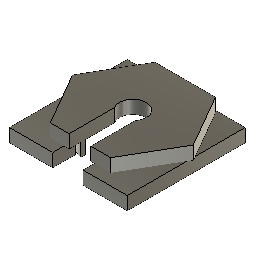
wall plug v1 v1 (Autodesk Fusion 360 design; units mm, degrees)
Autodesk Fusion 360 part; units mm, degrees
sketch "Sketch1" plane through (0, 0, 0) normal (0, 0, 1) x (1, 0, 0)
  line L0 (9.8948, 0) -> (0, 0)
  line L1 (0, 0) -> (0, 27)
  line L2 (0, 27) -> (27, 27)
  line L3 (27, 27) -> (27, 0)
  line L4 (27, 0) -> (16.8982, 0)
  circle A0 centre (13.6982, 15.0358) radius 10.55
  line L5 (9.8948, 0) -> (9.8948, 5.1952)
  line L6 (16.8982, 0) -> (16.8982, 4.9828)
  dimension "d1" = 27
  dimension "d2" = 27
  dimension "d3" = 21.1
  constraint coincident L0.end L1.start
  constraint horizontal L0
  constraint perpendicular L0 L1
  constraint perpendicular L1 L2
  constraint perpendicular L2 L3
  constraint perpendicular L3 L4
  constraint coincident A0 L5.end
  constraint perpendicular L0 L5
  constraint coincident A0 L6.end
  constraint perpendicular L4 L6
  measures "d1" distance of L0.end L1.end
  measures "d2" distance of L1.end L2.end
  measures "d3" diameter of A0
extrude "Extrude1" add sketch "Sketch1" along normal blind 3 contours L0 L1 L2 L3 L4 A0 L5 L6 makes body 1
sketch "Sketch2" plane through (0, 0, 0) normal (0, 0, 1) x (1, 0, 0)
  circle A0 centre (13.5664, 14.9736) radius 10
  dimension "d6" = 20
  measures "d6" diameter of A0
extrude "Extrude2" add sketch "Sketch2" along normal blind 3 separate body makes body 2
hole "Hole1" at (13.5664, 14.9736, 3) direction (0, 0, -1) diameter 18 depth 4 tip angle 118 bodies 2
sketch "Sketch3" plane through (0, 0, 3) normal (0, 0, 1) x (-1, 0, 0)
  circle A0 centre (-13.5664, -14.9736) radius 9
  circle A1 centre (-13.5664, -14.9736) radius 10
sketch "Sketch4" plane through (0, 0, 0) normal (0, 1, 0) x (1, 0, 0)
sketch "Sketch5" plane through (0, 0, 0) normal (0, 1, 0) x (1, 0, 0)
  line L0 (9, -3) -> (16, -3)
  line L1 (16, -3) -> (16, 0)
  line L2 (16, 0) -> (9, 0)
  line L3 (9, 0) -> (9, -3)
  constraint horizontal L0
  constraint vertical L1
  constraint horizontal L2
  constraint vertical L3
extrude "Extrude3" cut sketch "Sketch5" along normal blind 5 bodies 2
sketch "Sketch6" plane through (0, 0, 3) normal (0, 0, 1) x (-1, 0, 0)
  line L0 (-20.5886, -26.62) -> (-6.7322, -26.62)
  line L1 (-6.7322, -26.62) -> (0.196, -14.62)
  line L2 (0.196, -14.62) -> (-6.7322, -2.62)
  line L3 (-6.7322, -2.62) -> (-20.5886, -2.62)
  line L4 (-20.5886, -2.62) -> (-27.5168, -14.62)
  line L5 (-27.5168, -14.62) -> (-20.5886, -26.62)
  circle A0 centre (-13.6604, -14.62) radius 3.05
  point P0 (-13.6604, -14.62)
  dimension "d14" = 12
  dimension "d15" = 6.1
  constraint horizontal L0
  constraint coincident P0 A0.centre
  measures "d14" distance of P0 L5
  measures "d15" diameter of A0
extrude "Extrude4" add sketch "Sketch6" along normal blind 3 separate body makes body 3
sketch "Sketch7" plane through (0, 0, 0) normal (0, 1, 0) x (1, 0, 0)
  line L0 (11.05, -6) -> (16.0571, -6)
  line L1 (16.0571, -6) -> (16.0571, 0.7319)
  line L2 (16.0571, 0.7319) -> (11.05, 0.7319)
  line L3 (11.05, 0.7319) -> (11.05, -6)
  line L4 (11.05, 0.7319) -> (16.0571, 0.7319)
  constraint horizontal L0
  constraint vertical L1
  constraint horizontal L2
  constraint vertical L3
extrude "Extrude5" cut sketch "Sketch7" along normal blind 11 bodies 3 2 1
extrude "Extrude6" cut 1 faces at (12.719, 11, 4) along direction (0, 1, 0) blind 2 on bodies 3 bodies 3 2 1
combine "Combine1" operation add target body 2 tool bodies 3
